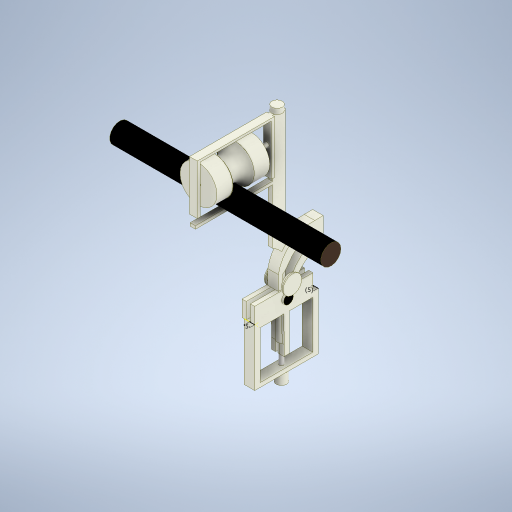
# Autodesk Inventor part: mechatronics
Saved by Autodesk Inventor 2024 (Build 280153000, 153)
## iProperties
Created: 2024-09-17
Part Number: mechatronics
Material: Generic
Document SubType Name: Modeling
Designer: manas
Density: 1 g/cm^3
Appearance: Smooth - Ivory
Author: manas
Autodesk Inventor part; units mm, degrees
sketch "Sketch1" plane through (0, 0, 0) normal (1, 0, 0) x (0, 1, 0)
  point P0 (0, 0)
sketch "Sketch2" plane through (0, 0, 0) normal (1, 0, 0) x (0, 1, 0)
  line L0 (-7.2773, 7.4258) -> (-11.2773, 7.4258)
  line L1 (-11.2773, 7.4258) -> (-11.2773, -52.5742)
  line L2 (-11.2773, -52.5742) -> (-7.2773, -52.5742)
  line L3 (-7.2773, -52.5742) -> (-7.2773, 7.4258)
  line L4 (-7.2773, 7.4258) -> (42.7227, 7.4258)
  line L5 (42.7227, 7.4258) -> (42.7227, 2.4258)
  line L6 (42.7227, 2.4258) -> (-7.2773, 2.4258)
  line L7 (-7.2773, 2.4258) -> (-7.2773, 7.4258)
  line L8 (-7.2773, -52.5742) -> (42.7227, -52.5742)
  line L9 (42.7227, -52.5742) -> (42.7227, -47.5742)
  line L10 (42.7227, -47.5742) -> (-7.2773, -47.5742)
  line L11 (-7.2773, -47.5742) -> (-7.2773, -52.5742)
  line L12 (42.7227, 2.4258) -> (37.7227, 2.4258)
  line L13 (37.7227, 2.4258) -> (37.7227, -47.5742)
  line L14 (37.7227, -47.5742) -> (42.7227, -47.5742)
  line L15 (42.7227, -47.5742) -> (42.7227, 2.4258)
  point P0 (0, 0)
  point P1 (-7.2773, -47.5742)
  point P2 (-7.2773, 2.4258)
  constraints: 32 end point, 8 parallel, 4 horizontal, 4 perpendicular, 1 point on line
extrude "Extrusion1" add sketch "Sketch2" along normal blind 10 contours L3 L2 L1 L0 | L4 L5 L6 L3 | L10 L9 L8 L3 | L6 L15 L10 L13
sketch "Sketch3" plane through (0, -11.2773, -52.5742) normal (0, -1, 0) x (1, 0, 0)
  point P0 (0, 52.5742)
sketch "Sketch4" plane through (0, -7.2773, 2.4258) normal (0, 1, 0) x (1, 0, 0)
  circle A0 centre (5, 25.2774) radius 2
  point P0 (0, 2.4258)
  dimension "d9" = 4
  constraints: 1 centre point
  measures "d9" diameter of A0
extrude "Extrusion2" add sketch "Sketch4" along normal blind 10
sketch "Sketch5" plane through (5, 2.7227, -22.8516) normal (0, 1, 0) x (1, 0, 0)
  circle A0 centre (0, 0) radius 2 projected
  circle A1 centre (0, 0) radius 2.5
  point P0 (-5, -22.8516)
  dimension "d12" = 5
  constraints: 1 centre point, 1 coincident
  measures "d12" diameter of A1
extrude "Extrusion3" add sketch "Sketch5" along normal blind 10 contours A0 | A1
sketch "Sketch6" plane through (5, 12.7227, -22.8516) normal (0, 1, 0) x (1, 0, 0)
  circle A0 centre (0, 0) radius 2 projected
  circle A1 centre (0, 0) radius 4
  point P0 (-5, -22.8516)
  dimension "d15" = 8
  constraints: 1 centre point, 1 coincident
  measures "d15" diameter of A1
extrude "Extrusion4" add sketch "Sketch6" along normal blind 30 contours A0 | A1
sketch "Sketch7" plane through (10, 0, 0) normal (1, 0, 0) x (0, 0, -1)
  line L0 (52.5742, 42.7227) -> (-7.4258, 42.7227) projected
  line L1 (-7.4258, 42.7227) -> (47.6868, 42.7227)
  line L2 (47.6868, 42.7227) -> (47.6868, 57.8367)
  line L3 (47.6868, 57.8367) -> (-7.4258, 57.8367)
  line L4 (-7.4258, 57.8367) -> (-7.4258, 42.7227)
  line L5 (-7.4258, 51.9066) -> (-7.4258, 99.2793) construction
  line L6 (-2.4258, 37.7227) -> (47.5742, 37.7227) projected
  line L7 (20.3516, 2.7227) -> (20.3516, 12.7227) projected
  line L8 (20.3516, 12.7227) -> (20.1305, 57.8367)
  line L9 (25.3516, 2.7227) -> (20.3516, 2.7227) projected
  line L10 (25.3516, 2.7227) -> (25.3516, 57.8367)
  line L11 (25.3516, 57.8367) -> (32.5832, 57.8367) construction
  line L12 (32.5832, 70.0782) -> (32.5832, 57.8367) construction
  arc A0 (32.5832, 57.8367) -> (32.5832, 57.8367) centre (32.5832, 2352.792) ccw
  line L13 (25.3516, 42.7227) -> (30.3516, 42.7227)
  line L14 (20.2046, 42.7227) -> (16.2046, 42.7227)
  line L15 (20.1305, 57.8367) -> (32.5832, 57.8367)
  line L16 (33.1718, 57.8367) -> (25.3516, 57.8367)
  line L17 (0, 90.3894) -> (0, 83.6146)
  line L18 (52.5742, 29257.2126) -> (52.5742, 29262.2126)
  line L19 (22.5742, 37.7227) -> (22.5742, 99.2793) construction
  line L20 (52.5742, 51.9066) -> (52.5742, 99.2793) construction
  line L21 (24.7968, 12.7227) -> (25.0179, 57.8367)
  line L22 (19.7968, 2.7227) -> (19.7968, 57.8367)
  arc A1 (45.1484, 83.6146) -> (25.0179, 57.8367) centre (51.7558, 57.7057) ccw
  arc A2 (45.1484, 90.3894) -> (19.7968, 57.8367) centre (53.3722, 57.8367) ccw
  arc A3 (52.5742, 78.4667) -> (30.035, 57.8367) centre (59.6559, 48.102) ccw
  arc A4 (52.5742, 99.2793) -> (11.9766, 57.8367) centre (53.5014, 57.7648) ccw
  line L23 (45.1484, 90.3894) -> (45.1484, 83.6146)
  line L24 (52.5742, 99.2793) -> (52.5742, 78.4667)
  point P0 (0, 0)
  point P1 (15.1135, 57.8367)
  point P2 (20.2046, 42.7227)
  point P3 (25.3516, 42.7227)
  dimension "d22" = 5
  dimension "d23" = 4
  dimension "d28" = 5
  constraints: 42 end point, 14 point on line, 10 point on circle, 10 symmetric about line, 5 centre point, 3 parallel, 3 vertical, 2 midpoint, 2 perpendicular, 1 collinear, 1 horizontal, 1 tangent
  measures "d22" distance of L13.start L13.end
  measures "d23" distance of L14.start L14.end
  measures "d28" distance of L18.start L18.end
extrude "Extrusion5" add sketch "Sketch7" against normal blind 4 contours L0 L10 L3 L2 | L10 L6 L21 L0 | L0 L21 L3 L10 | L21 L6 L8 L0 | L0 L8 L3 L21 | L10 L9 L7 L8 L6 | L0 L22 L3 L8 | L0 L4 L3 L22
sketch "Sketch8" plane through (0, 42.7227, 7.4258) normal (0, 1, 0) x (1, 0, 0)
  line L0 (10, 0) -> (5, 0)
  line L1 (0, 0) -> (6, 0) projected
  line L2 (6, 0) -> (6, 60)
  line L3 (0, 60) -> (0, 0) projected
  line L4 (0, 60) -> (10, 60) projected
  line L5 (10, 60) -> (5, 60)
  line L6 (5, 60) -> (5, 0)
  point P0 (0, 7.4258)
  dimension "d26" = 5
  dimension "d27" = 5
  constraints: 8 end point, 1 midpoint, 1 parallel, 1 point on line
  measures "d26" distance of L0.start L0.end
  measures "d27" distance of L4.end L5.end
sketch "Sketch9" plane through (6, 0, 0) normal (-1, 0, 0) x (0, 0, 1)
  point P0 (0, 0)
sketch "Sketch10" plane through (0, 42.7227, 7.4258) normal (0, 1, 0) x (1, 0, 0)
  point P0 (0, 7.4258)
ref_plane "Work Plane1" through (5, 42.7227, -52.5742) normal (0, 1, 0) x (0, 0, 1)
ref_plane "Work Plane2" through (4, 0, 0) normal (-1, 0, 0) x (0, 0, 1)
mirror "Mirror1" about plane through (4, 0, 0) normal (-1, 0, 0) of "Extrusion5"
sketch "Sketch11" plane through (-2, 78.4667, 7.4258) normal (-1, 0, 0) x (0, 0, 1)
  line L0 (-55.1125, -35.744) -> (0, -35.744) projected
  arc A0 (0, 20.8126) -> (-40.5976, -20.6299) centre (0.9272, -20.7018) ccw projected
  line L1 (-32.7774, -35.744) -> (-27.5462, -35.744)
  line L2 (-27.5462, -35.744) -> (-27.5462, 9.5236)
  line L3 (-27.5462, 9.5236) -> (-32.7774, 9.5236)
  line L4 (-32.7774, 9.5236) -> (-32.7774, -35.744)
  arc A1 (-7.4258, 5.1479) -> (-27.5563, -20.6299) centre (-0.8184, -20.761) ccw projected
  line L5 (-17.3274, 0.2719) -> (-27.5563, 0.2719)
  line L6 (-27.5563, 0.2719) -> (-27.5563, 100.2719)
  line L7 (-27.5563, 100.2719) -> (-17.3274, 100.2719)
  line L8 (-17.3274, 100.2719) -> (-17.3274, 0.2719)
  circle A2 centre (-30.1618, -23.5384) radius 2.6156
  point P0 (-7.4258, -78.4667)
  dimension "d30" = 100
  constraints: 16 end point, 4 parallel, 2 horizontal, 2 perpendicular, 2 point on circle, 1 centre point, 1 tangent
  measures "d30" distance of L5.end L6.end
extrude "Extrusion6" cut sketch "Sketch11" against normal through all contours A2
sketch "Sketch12" plane through (10, 0, 0) normal (1, 0, 0) x (0, 0, -1)
  circle A0 centre (22.595, 49.784) radius 2.8706
  point P0 (0, 0)
  constraints: 1 centre point
extrude "Extrusion7" add sketch "Sketch12" against normal blind 10
sketch "Sketch13" plane through (10, 0, 0) normal (1, 0, 0) x (0, 0, -1)
  arc A0 (21.7201, 52.518) -> (23.6183, 52.466) centre (22.595, 49.784) ccw projected
  circle A1 centre (22.595, 49.784) radius 4.6172
  point P0 (0, 0)
  point P1 (20.1625, 51.3081)
  point P2 (20.1775, 48.2361)
  constraints: 1 centre point, 1 coincident
extrude "Extrusion8" add sketch "Sketch13" along normal blind 2
sketch "Sketch14" plane through (0, 0, 0) normal (-1, 0, 0) x (0, 0, 1)
  arc A0 (-20.3638, 53.8263) -> (-25.0442, 53.698) centre (-22.595, 49.784) ccw projected
  circle A1 centre (-22.595, 49.784) radius 3.7479
  point P0 (0, 0)
  point P1 (-25.3516, 53.488)
  point P2 (-20.1507, 53.7011)
  constraints: 1 centre point, 1 coincident
extrude "Extrusion9" add sketch "Sketch14" along normal blind 2
sketch "Sketch15" plane through (-2, 78.4667, 7.4258) normal (-1, 0, 0) x (0, 0, 1)
  arc A0 (-29.1459, -25.9487) -> (-31.0441, -26.0007) centre (-30.0208, -28.6827) ccw projected
  circle A1 centre (-30.0208, -28.6827) radius 5.7276
  point P0 (-7.4258, -78.4667)
  point P1 (-27.6033, -30.2306)
  point P2 (-32.7774, -29.4837)
  constraints: 1 centre point, 1 coincident
extrude "Extrusion10" add sketch "Sketch15" along normal blind 2
sketch "Sketch16" plane through (4, 0, 0) normal (-1, 0, 0) x (0, 0, 1)
  line L0 (-52.5742, 42.7227) -> (-47.6868, 42.7227) projected
  arc A0 (7.4258, 99.2793) -> (-33.1718, 57.8367) centre (8.353, 57.7648) ccw projected
  line L1 (-20.2046, 42.7227) -> (-25.2981, 42.7227)
  line L2 (-25.2981, 42.7227) -> (-25.2981, 82.0942)
  line L3 (-25.2981, 82.0942) -> (-20.2046, 82.0942)
  line L4 (-20.2046, 82.0942) -> (-20.2046, 42.7227)
  line L5 (-25.2981, 82.0942) -> (-13.2981, 82.0942)
  line L6 (-13.2981, 82.0942) -> (-13.2981, 202.0942)
  line L7 (-13.2981, 202.0942) -> (-25.2981, 202.0942)
  line L8 (-25.2981, 202.0942) -> (-25.2981, 82.0942)
  point P0 (0, 0)
  point P1 (-25.3516, 42.7227)
  point P2 (-13.2981, 93.1985)
  dimension "d41" = 12
  dimension "d42" = 120
  constraints: 16 end point, 4 parallel, 2 horizontal, 2 perpendicular, 1 point on circle
  measures "d41" distance of L7.end L6.end
  measures "d42" distance of L6.end L5.end
extrude "Extrusion11" add sketch "Sketch16" along normal mid plane 4 contours A0 L8 L7 L6 | L3 L4 L1 L2
sketch "Sketch17" plane through (2, 202.0942, -25.2981) normal (0, 1, 0) x (1, 0, 0)
  line L0 (4, -5.5737) -> (0, -5.5737) projected
  circle A0 centre (2, -5.5737) radius 5
  point P0 (-2, -25.2981)
  dimension "d45" = 10
  constraints: 1 centre point, 1 midpoint
  measures "d45" diameter of A0
extrude "Extrusion12" add sketch "Sketch17" along normal blind 5
sketch "Sketch18" plane through (2, 202.0942, -13.2981) normal (0, 0, 1) x (1, 0, 0)
  line L0 (0, 0) -> (-3, 0) projected
  line L1 (-1.5, 0) -> (5.9013, 0)
  line L2 (5.9013, 0) -> (5.9013, -50)
  line L3 (5.9013, -50) -> (-1.5, -50)
  line L4 (-1.5, -50) -> (-1.5, 0)
  point P0 (-2, -202.0942)
  dimension "d52" = 50
  constraints: 8 end point, 2 parallel, 1 horizontal, 1 midpoint, 1 perpendicular
  measures "d52" distance of L1.end L2.end
extrude "Extrusion13" add sketch "Sketch18" along normal blind 3
sketch "Sketch19" plane through (2, 202.0942, -10.2981) normal (0, 0, 1) x (1, 0, 0)
  line L0 (-1.5, 0) -> (-1.5, -50) projected
  line L1 (5.9013, -50) -> (5.9013, 0) projected
  line L2 (-1.5, 0) -> (5.9013, 0)
  line L3 (5.9013, 0) -> (5.9013, -2.2124)
  line L4 (5.9013, -2.2124) -> (-1.5, -2.2124)
  line L5 (-1.5, -2.2124) -> (-1.5, 0)
  line L6 (4, -50) -> (5.9013, -50) projected
  line L7 (5.9013, -2.2124) -> (4.5229, -2.2124)
  line L8 (4.5229, -2.2124) -> (4.5229, -50)
  line L9 (4.5229, -50) -> (5.9013, -50)
  line L10 (5.9013, -50) -> (5.9013, -2.2124)
  line L11 (4.5229, -50) -> (-1.5, -50)
  line L12 (-1.5, -50) -> (-1.5, -12.1516)
  line L13 (-1.5, -12.1516) -> (4.5229, -12.1516)
  line L14 (4.5229, -12.1516) -> (4.5229, -50)
  line L15 (0, 0) -> (0, -120) projected
  line L16 (-1.5, -2.2124) -> (0, -2.2124)
  line L17 (0, -2.2124) -> (0, -12.1516)
  line L18 (0, -12.1516) -> (-1.5, -12.1516)
  line L19 (-1.5, -12.1516) -> (-1.5, -2.2124)
  line L20 (4.5229, -12.1516) -> (5.9013, -12.1516)
  point P0 (-2, -202.0942)
  point P1 (-1.5, -2.2124)
  constraints: 34 end point, 8 parallel, 6 point on line, 4 horizontal, 4 perpendicular
extrude "Extrusion14" add sketch "Sketch19" along normal blind 70 contours L2 L15 L4 L0 | L2 L1 L4 L15
sketch "Sketch20" plane through (0.5, 199.8817, -10.2981) normal (0, -1, 0) x (1, 0, 0)
  point P0 (-0.5, 10.2981)
sketch "Sketch21" plane through (2, 202.0942, -10.2981) normal (0, 0, 1) x (1, 0, 0)
  circle A0 centre (2, -23.3068) radius 2
  line L0 (4, -120) -> (4, 0) projected
  point P0 (-2, -202.0942)
  constraints: 1 centre point, 1 tangent
extrude "Extrusion15" add sketch "Sketch21" along normal blind 70
ref_plane "Work Plane3" through (2, 202.0942, 4.7019) normal (0, 0, 1) x (1, 0, 0)
sketch "Sketch22" plane through (2, 202.0942, 4.7019) normal (0, 0, 1) x (1, 0, 0)
  circle A0 centre (2, -23.3068) radius 2 projected
  circle A1 centre (2, -23.3068) radius 17.5
  point P0 (-2, -202.0942)
  dimension "d56" = 35
  constraints: 1 centre point, 1 coincident
  measures "d56" diameter of A1
extrude "Extrusion16" add sketch "Sketch22" along normal blind 15
ref_plane "Work Plane4" through (4, 178.7874, 39.7019) normal (0, 0, 1) x (1, 0, 0)
sketch "Sketch23" plane through (4, 178.7874, 39.7019) normal (0, 0, 1) x (1, 0, 0)
  circle A0 centre (0, 0) radius 17.5
  point P0 (-4, -178.7874)
  constraints: 1 centre point
extrude "Extrusion17" add sketch "Sketch23" along normal blind 15
ref_plane "Work Plane5" through (4.4013, 152.0942, -13.2981) normal (1, 0, 0) x (0, 0, -1)
sketch "Sketch24" plane through (4.4013, 152.0942, -13.2981) normal (1, 0, 0) x (0, 0, -1)
  line L0 (-53, 44.1932) -> (-53, 9.1932) projected
  line L1 (-33, 44.1932) -> (-33, 9.1932) projected
  arc A0 (-53, 44.1932) -> (-33, 44.1932) centre (-43, 48.0728) ccw
  arc A1 (-33, 9.1932) -> (-53, 9.1932) centre (-43, 8.272) ccw
  line L2 (-73, 28.6932) -> (-73, 24.6932) projected
  line L3 (-73, 26.6932) -> (-22.371, 26.6932)
  point P0 (-13.2981, -152.0942)
  point P1 (-53, 26.6932)
  point P2 (-33, 26.6932)
  constraints: 4 point on circle, 2 centre point, 2 end point, 1 horizontal, 1 midpoint
revolve "Revolution1" add sketch "Sketch24" angle 360 about axis through (4.4013, 178.7874, 59.7019) along (0, 0, -1) contours A0 L1 L3 L0
sketch "Sketch25" plane through (0.5, 199.8817, -10.2981) normal (0, -1, 0) x (1, 0, 0)
  line L0 (7.4013, -3) -> (7.4013, 70) projected
  line L1 (0, 0) -> (0, 70) projected
  line L2 (7.4013, 70) -> (0, 70)
  line L3 (0, 70) -> (0, 67.317)
  line L4 (0, 67.317) -> (7.4013, 67.317)
  line L5 (7.4013, 67.317) -> (7.4013, 70)
  point P0 (-0.5, 10.2981)
  constraints: 8 end point, 2 parallel, 1 horizontal, 1 perpendicular, 1 point on line
extrude "Extrusion18" add sketch "Sketch25" along normal blind 45
sketch "Sketch26" plane through (6, 0, 0) normal (1, 0, 0) x (0, 0, -1)
  line L0 (25.2981, 202.0942) -> (25.2981, 82.0942) projected
  line L1 (25.2981, 145.1687) -> (-59.5491, 145.1687)
  line L2 (-59.5491, 145.1687) -> (-59.5491, 148.0219)
  line L3 (-59.5491, 148.0219) -> (25.2981, 148.0219)
  line L4 (25.2981, 148.0219) -> (25.2981, 145.1687)
  line L5 (-17.1255, 145.1687) -> (-1.3841, 92.9414)
  line L6 (-22.4809, 145.1687) -> (-6.2935, 91.4617)
  line L7 (-6.2935, 91.4617) -> (-1.3841, 92.9414)
  point P0 (0, 0)
  constraints: 14 end point, 3 parallel, 2 perpendicular, 2 point on line, 1 horizontal, 1 midpoint
extrude "Extrusion19" add sketch "Sketch26" against normal blind 5 contours L0 L1 L2 L3
sketch "Sketch27" plane through (6, 0, 0) normal (1, 0, 0) x (0, 0, -1)
  line L0 (-59.5491, 145.1687) -> (13.2981, 145.1687) projected
  arc A0 (-23.1255, 145.1687) -> (-31.9958, 145.1687) centre (-27.5606, 135.0964) ccw
  line L1 (-16.0659, 145.1687) -> (40.1629, 87.9908)
  line L2 (40.1629, 87.9908) -> (34.1667, 82.0942)
  line L3 (34.1667, 82.0942) -> (-27.8608, 145.1687)
  line L4 (-27.8608, 145.1687) -> (-16.0659, 145.1687)
  line L5 (25.2981, 145.1687) -> (25.2981, 82.0942) projected
  point P0 (0, 0)
  constraints: 8 end point, 3 perpendicular, 3 point on line, 2 point on circle, 1 centre point, 1 midpoint
extrude "Extrusion20" [suppressed]
mirror "Mirror2" [suppressed]
sketch "Sketch28" plane through (4.4013, 152.0942, -13.2981) normal (1, 0, 0) x (0, 0, -1)
  circle A0 centre (-43, 6.5802) radius 9.5258
  point P0 (-13.2981, -152.0942)
  constraints: 1 centre point
extrude "Extrusion21" add sketch "Sketch28" along normal mid plane 200
sketch "Sketch29" plane through (0, -11.2773, -52.5742) normal (0, -1, 0) x (1, 0, 0)
  circle A0 centre (5, 29.7226) radius 2 projected
  circle A1 centre (5, 29.7226) radius 5
  point P0 (0, 52.5742)
  dimension "d72" = 10
  constraints: 1 centre point, 1 coincident
  measures "d72" diameter of A1
extrude "Extrusion22" add sketch "Sketch29" along normal blind 10 contours A0 | A1
sketch "Sketch30" plane through (4, 0, 0) normal (-1, 0, 0) x (0, 0, 1)
  point P0 (0, 0)
sketch "Sketch31" plane through (4, 0, 0) normal (-1, 0, 0) x (0, 0, 1)
  line L0 (-20.2046, 42.7227) -> (-20.3516, 12.7227) projected
  line L1 (-20.2046, 42.7227) -> (-20.2046, 82.0942)
  arc A0 (-25.103, 75.3384) -> (-50.4081, 91.3683) centre (-53.9195, 57.8367) ccw
  arc A1 (-25.2981, 57.8367) -> (-50.4081, 84.5944) centre (-68.3177, 42.6269) ccw
  line L2 (7.4258, 57.8367) -> (-20.2046, 57.8367) projected
  line L3 (-15.9358, 57.8367) -> (-15.9358, 71.6374)
  arc A2 (-15.9358, 71.6374) -> (-50.4081, 98.8368) centre (-48.7286, 65.5206) ccw
  line L4 (-47.6868, 57.8367) -> (7.4258, 57.8367) projected
  arc A3 (-31.6698, 57.8367) -> (-58.4509, 77.5803) centre (-63.72, 42.3977) ccw
  line L5 (-58.1905, 97.5091) -> (-58.1905, 97.5091)
  line L6 (-58.4509, 98.8368) -> (-58.4509, 77.5803)
  arc A4 (-58.4509, 77.5803) -> (-58.4509, 77.5803) centre (-97.6953, 77.5803) ccw
  line L7 (-58.4509, 77.5803) -> (-58.4509, 98.8368)
  line L8 (-50.4081, 98.8368) -> (-58.4509, 98.8368)
  line L9 (-50.4081, 91.3683) -> (-50.4081, 84.5944)
  line L10 (-20.2046, 57.8367) -> (-20.2046, 70.0254)
  arc A5 (-20.6498, 69.647) -> (-20.2046, 70.0254) centre (-25.103, 75.3384) ccw
  line L11 (-20.2046, 63.9311) -> (-20.2046, 57.8367)
  arc A6 (-20.6498, 69.647) -> (-20.2046, 70.0254) centre (-25.103, 75.3384) ccw
  line L12 (-20.2046, 70.0254) -> (-20.2046, 57.8367)
  arc A7 (-25.103, 75.3384) -> (-20.2046, 70.0254) centre (-9.4827, 84.8254) ccw
  line L13 (-20.2046, 57.8367) -> (-20.2046, 82.0942) projected
  line L14 (-20.2046, 70.0254) -> (-20.2046, 57.8367)
  line L15 (-20.2046, 57.8367) -> (-25.2981, 57.8367)
  point P0 (0, 0)
  constraints: 24 end point, 16 point on circle, 8 centre point, 4 point on line, 3 collinear, 3 tangent, 3 vertical, 2 coincident, 1 horizontal, 1 midpoint, 1 perpendicular
extrude "Extrusion23" add sketch "Sketch31" along normal mid plane 10 contours L1 A7 A0 L9 A1 L4 A3 L6 L8 A2 L3 L2
sketch "Sketch32" plane through (4, 0, 0) normal (-1, 0, 0) x (0, 0, 1)
  line L0 (59.5491, 145.1687) -> (-13.2981, 145.1687) projected
  line L1 (8.702, 145.1687) -> (-25.2981, 107.3561)
  line L2 (-25.2981, 89.265) -> (-25.2981, 202.0942) projected
  line L3 (-21.1745, 99.3978) -> (19.9815, 145.1687)
  line L4 (19.9815, 145.1687) -> (8.702, 145.1687)
  line L5 (-21.1745, 99.3978) -> (-25.2981, 107.3561)
  point P0 (0, 0)
  constraints: 8 end point, 2 point on line, 1 parallel, 1 perpendicular
extrude "Extrusion24" add sketch "Sketch32" along normal mid plane 10
sketch "Sketch33" plane through (-2, 2.7227, -25.3516) normal (-1, 0, 0) x (0, 0, 1)
  line L0 (0.0535, 55.114) -> (0.0535, 72.9329) projected
  circle A0 centre (0.0535, 58.857) radius 7.3567
  point P0 (25.3516, -2.7227)
  constraints: 1 centre point, 1 point on line
extrude "Extrusion25" add sketch "Sketch33" along normal blind 2
sketch "Sketch34" plane through (-4, 78.4667, 7.4258) normal (-1, 0, 0) x (0, 0, 1)
  line L0 (-38.3791, -33.1716) -> (-21.6626, -33.1716)
  line L1 (-21.6626, -33.1716) -> (-21.6626, -24.1938)
  line L2 (-21.6626, -24.1938) -> (-38.3791, -24.1938)
  line L3 (-38.3791, -24.1938) -> (-38.3791, -33.1716)
  arc A0 (-33.5782, -24.1938) -> (-27.5462, -23.5173) centre (-30.0208, -28.6827) ccw projected
  line L4 (-38.3791, -33.1716) -> (-21.6626, -24.1938) construction
  line L5 (-21.6626, -33.1716) -> (-38.3791, -24.1938) construction
  point P0 (-7.4258, -78.4667)
  point P1 (-26.4634, -24.1938)
  constraints: 12 end point, 2 midpoint, 2 parallel, 1 horizontal, 1 perpendicular
extrude "Extrusion26" cut sketch "Sketch34" against normal blind 2 contours A0 L2 L0 | L0 A0
sketch "Sketch35" plane through (-4, 78.4667, 7.4258) normal (-1, 0, 0) x (0, 0, 1)
  line L0 (-32.7239, -20.6299) -> (-32.7239, -2.8111) projected
  circle A0 centre (-32.7239, -17.616) radius 8.8017
  point P0 (-7.4258, -78.4667)
  constraints: 1 centre point, 1 point on line
extrude "Extrusion27" add sketch "Sketch35" along normal blind 1
mirror "Mirror3" about plane through (4, 0, 0) normal (-1, 0, 0) of "Extrusion27", "Extrusion25"
body "Solid1"
